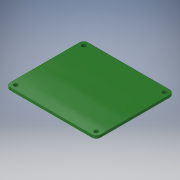
# Autodesk Inventor part: Pi Foundation Display Driver Board
Saved by Autodesk Inventor 2017 SP1 (Build 210196100, 196)
## iProperties
Part Number: Pi Foundation Display Driver Board
Material: Generisch
Document SubType Name: Modeling
Designer: u26048
Density: 1 g/cm^3
Appearance: Waldgrün
Author: u26048
Autodesk Inventor part; units mm, degrees
ref_plane "YZ Plane" through (0, 0, 0) normal (1, 0, 0) x (0, 1, 0)
ref_plane "XZ Plane" through (0, 0, 0) normal (0, 1, 0) x (-1, 0, 0)
ref_plane "XY Plane" through (0, 0, 0) normal (0, 0, 1) x (1, 0, 0)
sketch "Skizze1" plane through (0, 0, 0) normal (0, 0, 1) x (1, 0, 0)
  line L0 (-29.5, 28) -> (29.5, 28)
  line L1 (32.5, 25) -> (32.5, -25)
  line L2 (29.5, -28) -> (-29.5, -28)
  line L3 (-32.5, -25) -> (-32.5, 25)
  arc A0 (-29.5, 28) -> (-32.5, 25) centre (-29.5, 25) ccw
  arc A1 (-32.5, -25) -> (-29.5, -28) centre (-29.5, -25) ccw
  arc A2 (29.5, -28) -> (32.5, -25) centre (29.5, -25) ccw
  arc A3 (32.5, 25) -> (29.5, 28) centre (29.5, 25) ccw
  line L4 (-29, 24.5) -> (29, 24.5) construction
  line L5 (29, 24.5) -> (29, -24.5) construction
  line L6 (29, -24.5) -> (-29, -24.5) construction
  line L7 (-29, -24.5) -> (-29, 24.5) construction
  circle A4 centre (-29, 24.5) radius 1.375
  circle A5 centre (29, 24.5) radius 1.375
  circle A6 centre (-29, -24.5) radius 1.375
  circle A7 centre (29, -24.5) radius 1.375
  point P0 (0, 0)
  point P1 (32.5, -28)
  point P2 (32.5, 28)
  point P3 (-32.5, -28)
  point P4 (0, 28)
  point P5 (32.5, 0)
  point P6 (0, 24.5)
  point P7 (29, 0)
  dimension "d0" = 65
  dimension "d1" = 56
  dimension "d2" = 3
  dimension "d3" = 58
  dimension "d4" = 49
  dimension "d5" = 2.75
  dimension "d8" = 58
  dimension "d11" = 49
  constraints: 16 end point, 8 centre point, 8 point on circle, 8 tangent, 6 point on line, 5 coincident, 4 midpoint, 4 parallel, 3 equal radius, 3 horizontal, 2 horizontal alignment, 2 perpendicular, 2 vertical alignment, 1 vertical, 9 other
  measures "d0" distance of point (32.5, -28) point (-32.5, -28)
  measures "d1" distance of point (32.5, 28) point (32.5, -28)
  measures "d2" radius of A0
  measures "d3" distance of L5.end L6.end
  measures "d4" distance of L4.end L5.end
  measures "d5" diameter of A4
  measures "d8" distance of A4.centre A5.centre
  measures "d11" distance of A4.centre A6.centre
extrude "Extrusion1" add sketch "Skizze1" along normal blind 1.75
